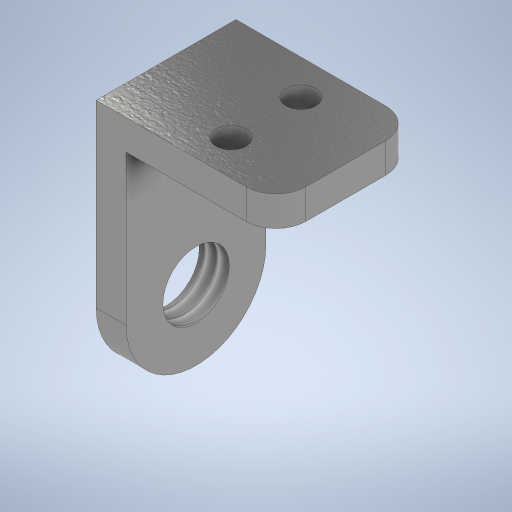
# Autodesk Inventor part: HUDSON-1-77
Saved by Autodesk Inventor 2024.2 (Build 282272000, 272)
## iProperties
Created: 2024-09-29
Part Number: HUDSON-1-77
Material: Generic
Document SubType Name: Modeling
Designer: melim
Density: 1 g/cm^3
Appearance: Galvanized
Author: melim
Autodesk Inventor part; units mm, degrees
ref_plane "YZ Plane" through (0, 0, 0) normal (1, 0, 0) x (0, 1, 0)
ref_plane "XZ Plane" through (0, 0, 0) normal (0, 1, 0) x (-1, 0, 0)
ref_plane "XY Plane" through (0, 0, 0) normal (0, 0, 1) x (1, 0, 0)
sketch "Sketch1" plane through (0, 0, 0) normal (0, 0, 1) x (1, 0, 0)
  line L0 (0, 0) -> (0, 25)
  line L1 (0, 25) -> (18, 25)
  line L2 (18, 25) -> (18, 22)
  line L3 (18, 22) -> (3, 22)
  line L4 (3, 22) -> (3, 0)
  line L5 (3, 0) -> (0, 0)
  dimension "d0" = 25
  dimension "d1" = 3
  dimension "d2" = 3
  dimension "d3" = 15
  constraints: 12 end point, 4 perpendicular, 1 horizontal, 1 vertical
  measures "d0" distance of L0.start L0.end
  measures "d1" distance between parallel lines of L0 L4
  measures "d2" distance between parallel lines of L3 L1
  measures "d3" distance of L2.end L3.end
extrude "Extrusion1" add sketch "Sketch1" along normal blind 14
fillet "Fillet1" radius 7 2 edges at (1.5, 0, 14) (1.5, 0, 0)
sketch "Sketch2" plane through (3, 22, 14) normal (1, 0, 0) x (0, 0, -1)
  line L0 (14, 3) -> (0, 3) projected
  line L1 (0, -15) -> (0, 0) projected
  arc A0 (0, -15) -> (14, -15) centre (7, -15) ccw projected
  line L2 (14, -15) -> (14, 0) projected
  line L3 (14, 0) -> (0, 0) projected
  line L4 (0, -15) -> (0, 0) projected
  point P0 (14, -22)
  point P1 (7, -15)
  dimension "d7" = 18
  dimension "d8" = 7
  measures "d7" distance from line of L0 point (7, -15)
  measures "d8" distance from line of L1 point (7, -15)
hole "Hole1" at (3, 7, 7) direction (-1, 0, 0) diameter 6.647 end through all thread size "M8x1.25" class "6H" standard "ANSI Metric M Profile"
sketch "Sketch3" plane through (0, 25, 0) normal (0, 1, 0) x (1, 0, 0)
  line L0 (18, -14) -> (0, -14) projected
  line L1 (0, 0) -> (0, -14) projected
  point P0 (10, -10.5)
  point P1 (10, -3.5)
  dimension "d16" = 7
  dimension "d17" = 3.5
  dimension "d18" = 10
  dimension "d19" = 10
  measures "d16" distance of point (10, -10.5) point (10, -3.5)
  measures "d17" distance from line of L0 point (10, -10.5)
  measures "d18" distance from line of L1 point (10, -10.5)
  measures "d19" distance from line of L1 point (10, -3.5)
hole "Hole2" at (10, 25, 10.5) at (10, 25, 3.5) direction (0, -1, 0) diameter 3 end through all
fillet "Fillet2" radius 3 2 edges at (18, 23.5, 0) (18, 23.5, 14)
body "Solid1"
